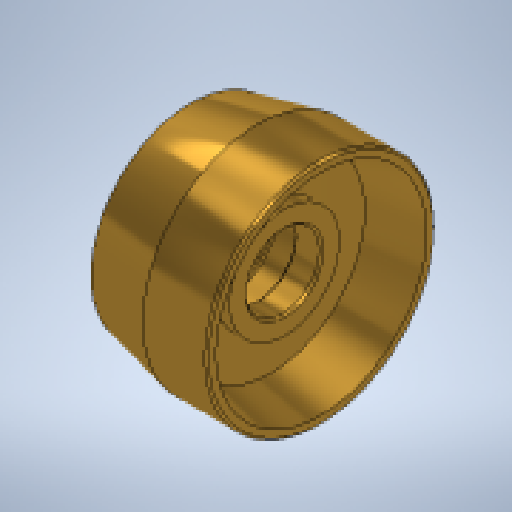
# Autodesk Inventor part: Flywheel
Saved by Autodesk Inventor 2023.2 (Build 272271000, 271)
## iProperties
Created: 2024-01-10
Part Number: Flywheel
Material: Brass, Soft Yellow
Document SubType Name: Modeling
Designer: Nathan Cai
Mass: 213.55 g
Surface Area: 103.86 cm^2
Volume: 25.2125 cm^3
Density: 8.47 g/cm^3
Appearance: Brass - Satin
Author: Nathan Cai
Autodesk Inventor part; units mm, degrees
ref_plane "YZ Plane" through (0, 0, 0) normal (1, 0, 0) x (0, 1, 0)
ref_plane "XZ Plane" through (0, 0, 0) normal (0, 1, 0) x (-1, 0, 0)
ref_plane "XY Plane" through (0, 0, 0) normal (0, 0, 1) x (1, 0, 0)
sketch "Sketch1" plane through (0, 0, 0) normal (0, 1, 0) x (-1, 0, 0)
  line L0 (0, 0) -> (1, 0)
  line L1 (1, 0) -> (1, -8)
  line L2 (1, -8) -> (0, -8)
  line L3 (0, -8) -> (0, 0)
  line L4 (1, 0) -> (11.5, 0)
  line L5 (11.5, 0) -> (11.5, -14)
  line L6 (11.5, -14) -> (1, -14)
  line L7 (1, -14) -> (1, 0)
  line L8 (0, 0) -> (-13, 0)
  line L9 (-13, 0) -> (-13, -25)
  line L10 (-13, -25) -> (0, -25)
  line L11 (0, -25) -> (0, 0)
  line L12 (-13, -23) -> (0, -20.118)
  line L13 (-13, 0) -> (11.5, 0)
  line L14 (11.5, 0) -> (11.5, -25)
  line L15 (11.5, -25) -> (-13, -25)
  line L16 (-13, -25) -> (-13, 0)
  line L17 (-13, -25) -> (0, -22.118) construction
  line L18 (11.5, -25) -> (15.5, -25)
  line L19 (15.5, -25) -> (15.5, -18.5)
  line L20 (15.5, -18.5) -> (11.5, -18.5)
  line L21 (11.5, -18.5) -> (11.5, -25)
  line L22 (0, -8) -> (-5, -8)
  line L23 (-5, -8) -> (-5, -12)
  line L24 (-5, -12) -> (0, -12)
  line L25 (0, -12) -> (0, -8)
  line L26 (1, -8) -> (-2, -8)
  line L27 (-2, -8) -> (-2, -25)
  line L28 (-2, -25) -> (1, -25)
  line L29 (1, -25) -> (1, -8)
  line L30 (1, -25) -> (15.5, -21.7854)
  point P0 (1, -8)
  point P1 (0, -8)
  point P2 (0, -25)
  point P3 (11.5, -18.5)
  point P4 (0, -12)
  point P5 (0, -8)
  point P6 (0, -25)
  point P7 (-2, -12)
  point P8 (-2, -20.5614)
  point P9 (1, -25)
  dimension "d0" = 1
  dimension "d1" = 8
  dimension "d2" = 10.5
  dimension "d3" = 14
  dimension "d6" = 13
  dimension "d7" = 25
  dimension "d9" = 23
  dimension "d35" = 4
  dimension "d36" = 18.5
  dimension "d41" = 4
  dimension "d42" = 12.5
  dimension "d43" = 6
  dimension "d44" = 3
  constraints: 62 end point, 16 parallel, 7 horizontal, 7 perpendicular, 7 point on line
  measures "d0" distance of L1.end L2.end
  measures "d1" distance of L0.end L1.end
  measures "d2" distance of L5.end L6.end
  measures "d3" distance of L4.end L5.end
  measures "d6" distance of L10.end L9.end
  measures "d7" distance of L9.end L8.end
  measures "d9" distance from line of L8 L12.start
  measures "d35" distance of L20.end L19.end
  measures "d36" distance between parallel lines of L8 L20
  measures "d41" distance of L23.end L22.end
  measures "d42" angle of L15 L12
  measures "d43" distance between parallel lines of L7 L23
  measures "d44" distance between parallel lines of L29 L27
revolve "Revolution1" add sketch "Sketch1" angle 360 about axis through (0, 0, 0) along (-1, 0, 0) contours L2 L7 L29 L15 L11 | L11 L24 L27 L22 | L11 L12 L27 L24 | L27 L24 L23 L22 | L12 L27 L10 L9 | L6 L14 L30 L29 | L11 L10 L27 L12 | L20 L19 L30 L14
chamfer "Chamfer2" distance 0.5 angle 45 2 edges at (-1, 0, 8) (5, 0, 8)
chamfer "Chamfer4" distance 0.5 angle 45 1 edges at (13, 0, 25)
chamfer "Chamfer5" distance 2 angle 45 1 edges at (-11.5, 0, 14)
body "Solid1"
